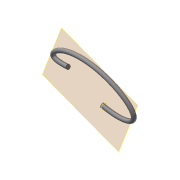
# Autodesk Inventor part: Wire to Spark Gap 2
Saved by Autodesk Inventor 2018 (Build 220112000, 112)
## iProperties
Created: 2018-08-02
Part Number: Wire to Spark Gap 2
Material: Generic
Document SubType Name: Modeling
Designer: DPLXuser
Density: 1 g/cm^3
Appearance: Default
Author: DPLXuser
Autodesk Inventor part; units mm, degrees
ref_plane "YZ Plane" through (0, 0, 0) normal (1, 0, 0) x (0, 1, 0)
ref_plane "XZ Plane" through (0, 0, 0) normal (0, 1, 0) x (-1, 0, 0)
ref_plane "XY Plane" through (0, 0, 0) normal (0, 0, 1) x (1, 0, 0)
ref_plane "Work Plane1" through (180.6657, -103.4431, 58.8853) normal (0, -0.1058, 0.9944) x (0.4079, 0.9079, 0.0966)
sketch "Sketch1" plane through (180.6657, -103.4431, 58.8853) normal (0, -0.1058, 0.9944) x (0.4079, 0.9079, 0.0966)
  line L0 (-1.7341, 3.8684) -> (7.2859, -47.1153) construction
  line L1 (7.2859, -47.1153) -> (50.0533, -72.8947) construction
  line L2 (50.0533, -72.8947) -> (88.6228, -47.1153) construction
  line L3 (88.6228, -47.1153) -> (96.3512, 29.555) construction
  line L4 (96.3512, 29.555) -> (71.8704, 102.8109) construction
  line L5 (71.8704, 102.8109) -> (52.1284, 161.8867) construction
  line L6 (52.1284, 161.8867) -> (-20.4224, 179.4685) construction
  line L7 (-20.4224, 179.4685) -> (10.4433, 110.9284) construction
  spline S0 degree 4 poles (-1.7341, 3.8684) (7.2859, -47.1153) (50.0533, -72.8947) (88.6228, -47.1153) (96.3512, 29.555) (71.8704, 102.8109) (52.1284, 161.8867) (-20.4224, 179.4685) (10.4433, 110.9284) knots 1 1 1 1 1 2 3 4 5 6 6 6 6 6
  point P0 (14.5265, 204.3684)
  constraints: 3 other
ref_plane "Work Plane2" through (180.6657, -103.4431, 58.8853) normal (1, 0, 0) x (0, 0.9996, 0.0291)
sketch "Sketch2" plane through (180.6657, -103.4431, 58.8853) normal (1, 0, 0) x (0, 0.9996, 0.0291)
  circle A0 centre (0, 0) radius 6.35
  point P0 (101.6845, -61.8726)
  dimension "d0" = 12.7
  constraints: 1 centre point
  measures "d0" diameter of A0
sweep "Sweep1" add profiles "Sketch2" path "Sketch1"
body "Solid1"
